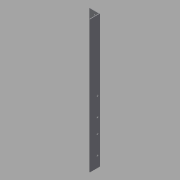
# Autodesk Inventor part: 26in Angle Channel CIM Mount Left
Saved by Autodesk Inventor 2013 (Build 170138000, 138)
## iProperties
Created: 2013-01-27
Part Number: 26in Angle Channel CIM Mount Left
Material: Aluminum 6061
Document SubType Name: Modeling
Designer: Naphat
Density: 1 g/cm^3
Author: Naphat
Autodesk Inventor part; units mm, degrees
ref_plane "YZ Plane" through (0, 0, 0) normal (1, 0, 0) x (0, 1, 0)
ref_plane "XZ Plane" through (0, 0, 0) normal (0, 1, 0) x (-1, 0, 0)
ref_plane "XY Plane" through (0, 0, 0) normal (0, 0, 1) x (1, 0, 0)
sketch "Sketch1" plane through (0, 0, 0) normal (0, 1, 0) x (-1, 0, 0)
  line L0 (0, 0) -> (50, 0)
  line L1 (50, 0) -> (50, 3)
  line L2 (0, 0) -> (0, 50)
  line L3 (0, 50) -> (3, 50)
  line L4 (3, 50) -> (3, 3)
  line L5 (3, 3) -> (50, 3)
  dimension "d0" = 50
  dimension "d1" = 3
  dimension "d2" = 50
  dimension "d3" = 3
  constraints: 12 end point, 3 perpendicular, 2 parallel, 1 horizontal
  measures "d0" distance of L0.start L0.end
  measures "d1" distance of L0.end L1.end
  measures "d2" distance of L0.start L2.end
  measures "d3" distance of L2.end L3.end
extrude "Extrusion1" add sketch "Sketch1" along normal blind 660.4
sketch "Sketch4" plane through (0, 0, 0) normal (0, 0, -1) x (-1, 0, 0)
  circle A0 centre (25, 15.7) radius 3.175
  circle A1 centre (25, 644.7) radius 3.175
  dimension "d62" = 6.35
  dimension "d63" = 6.35
  constraints: 2 centre point
  measures "d62" diameter of A0
  measures "d63" diameter of A1
extrude "Extrusion4" cut sketch "Sketch4" against normal blind 25.4
sketch "Sketch5" plane through (-3, 0, 3) normal (-1, 0, 0) x (0, 0, 1)
  circle A0 centre (9.7942, 55.1) radius 5
  circle A1 centre (9.7942, 148.1) radius 5
  circle A2 centre (9.7942, 220.2) radius 5
  circle A3 centre (9.7942, 313.2) radius 5
  point P0 (-3, 0)
  constraints: 4 centre point
extrude "Extrusion5" cut sketch "Sketch5" against normal blind 25.4
equation "\"d63\" = d62"
body "Solid1"
